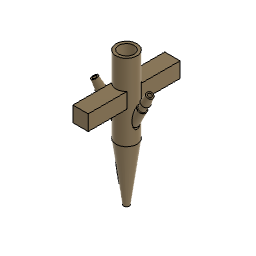
Flush_tool v11 (Autodesk Fusion 360 design; units mm, degrees)
Autodesk Fusion 360 part; units mm, degrees
note: some values were not read from the file. Chosen so that the rebuilt part matches the saved one: where a step starts.
sketch "Sketch1" plane through (0, 0, 0) normal (0, 0, 1) x (1, 0, 0)
  circle A0 centre (0, 0) radius 4
  circle A1 centre (0, 0) radius 5.5
  dimension "d1" = 8
  dimension "d2" = 11
  constraint coincident A0.centre A1.centre
  measures "d1" diameter of A0
  measures "d2" diameter of A1
ref_plane "WorkPlane1" through (0, 0, -15) normal (0, 0, 1) x (1, 0, 0)
sketch "Sketch2" plane through (0, 0, -15) normal (0, 0, 1) x (1, 0, 0)
  circle A0 centre (0, 0) radius 3.45
  dimension "d6" = 6.9
  constraint coincident A0.centre origin
  measures "d6" diameter of A0
extrude "Extrude1" add sketch "Sketch1" against normal blind 40 contours A0 | A1
ref_plane "WorkPlane2" through (0, 0, -70) normal (0, 0, -1) x (-1, 0, 0)
sketch "Sketch3" plane through (0, 0, -70) normal (0, 0, -1) x (-1, 0, 0)
  circle A0 centre (0, 0) radius 1.5
  dimension "d10" = 3
  constraint coincident A0.centre origin
  measures "d10" diameter of A0
loft "Loft1" add profiles "Sketch3" section 1 face at (-1.4907, 0.2732, -40) section 2
ref_plane "WorkPlane3" through (0, 0, 0) normal (0, 1, 0) x (0, 0, 1)
sketch "Sketch4" plane through (0, 0, 0) normal (0, 1, 0) x (1, 0, 0)
  line L0 (0, 0) -> (0, 15) construction
  line L1 (0, 15) -> (4, 15)
  line L2 (0, 15) -> (-4, 15)
  line L3 (-4, 15) -> (-4, 23)
  line L4 (-4, 23) -> (4, 23)
  line L5 (4, 23) -> (4, 15)
  dimension "d12" = 15
  dimension "d13" = 4
  dimension "d14" = 4
  dimension "d15" = 8
  dimension "d16" = 8
  dimension "d17" = 8
  constraint coincident L0.start origin
  constraint vertical L0
  constraint horizontal L1
  constraint perpendicular L0 L2
  constraint perpendicular L2 L3
  constraint perpendicular L3 L4
  constraint perpendicular L4 L5
  measures "d12" distance of L0.start L0.end
  measures "d13" distance of L0.end L1.end
  measures "d14" distance of L0.end L2.end
  measures "d15" distance of L2.end L3.end
  measures "d16" distance of L3.end L4.end
  measures "d17" distance of L4.end L1.end
extrude "Extrude2" add sketch "Sketch4" along normal blind 24 and the other way blind 24
loft "Loft2" cut profiles "Sketch1", "Sketch2" section 1 contours A0 section 2
extrude "Extrude3" cut sketch "Sketch2" against normal blind 3
ref_plane "WorkPlane4" through (0, 0, -28) normal (0, 0, 1) x (1, 0, 0)
sketch "Sketch5" plane through (0, 0, -28) normal (0, 0, 1) x (1, 0, 0)
  circle A0 centre (0, 0) radius 5.5
  line L0 (0, 0) -> (5.5, 0)
  line L1 (0, 0) -> (-4.7631, -2.75)
  line L2 (0, 0) -> (5.5, 0) construction
  line L3 (0, 0) -> (-4.7631, 2.75)
  line L4 (0, 0) -> (5.5, 0) construction
  line L5 (0, 0) -> (4.7631, -2.75) construction
  line L6 (0, 0) -> (5.5, 0) construction
  line L7 (0, 0) -> (4.7631, 2.75) construction
  line L8 (0, 0) -> (5.5, 0) construction
  dimension "d25" = 150
  dimension "d26" = 5.5
  dimension "d27" = 150
  dimension "d28" = 5.5
  dimension "d29" = 5.5
  dimension "d30" = 30
  dimension "d32" = 5.5
  dimension "d33" = 30
  constraint coincident A0.centre L0.start
  constraint coincident A0 L0.end
  constraint horizontal L0
  constraint horizontal L2
  constraint horizontal L4
  constraint horizontal L6
  constraint horizontal L8
  measures "d25" angle of L1 L2
  measures "d26" distance of A0.centre L1.end
  measures "d27" angle of L3 L4
  measures "d28" distance of A0.centre L3.end
  measures "d29" distance of A0.centre L5.end
  measures "d30" angle of L5 L6
  measures "d32" distance of A0.centre L7.end
  measures "d33" angle of L7 L8
ref_plane "WorkPlane5" through (-4.7631, -2.75, -28) normal (-0.5, 0.866025, 0) x (-0.866025, -0.5, 0)
sketch "Sketch6" plane through (0, 0, 0) normal (-0.5, 0.866025, 0) x (-0.866025, -0.5, 0)
  line L0 (-5.5, -40) -> (5.5, -40) construction
  line L1 (-5.5, -40) -> (5.5, -40) construction
  line L2 (1.5, -70) -> (-1.5, -70) construction
  line L3 (5.5, -40) -> (2.5, -40) construction
  line L4 (5.5, -28) -> (2.5, -28) construction
  line L5 (2.5, -28) -> (2.5, -33.991) construction
  line L6 (5.5, -28) -> (2.5, -33.991) construction
  line L7 (2.5, -40) -> (2.5, -33.991) construction
  line L8 (-5.5, -23) -> (-15.4641, -23)
  line L9 (-15.4641, -15) -> (-15.4641, -23)
  line L10 (-5.5, -15) -> (-15.4641, -15)
  line L11 (8.5359, -15) -> (15.4641, -15)
  line L12 (8.5359, -15) -> (5.5, -15)
  line L13 (15.4641, -15) -> (15.4641, -23)
  line L14 (15.4641, -23) -> (8.5359, -23)
  line L15 (8.5359, -23) -> (5.5, -23)
  line L16 (1.5, -70) -> (-1.5, -70)
  line L17 (5.5, 0) -> (-5.5, 0)
  line L18 (1.5, -70) -> (5.5, -40)
  line L19 (-1.5, -70) -> (-5.5, -40)
  line L20 (-5.5, 0) -> (-5.5, -15)
  line L21 (-5.5, -23) -> (-5.5, -40)
  line L22 (5.5, 0) -> (5.5, -15)
  line L23 (5.5, -23) -> (5.5, -40)
  line L24 (5.5, -28) -> (12.2164, -14.5877)
  line L25 (5.5, -28) -> (15.5, -28) construction
  line L26 (5.5, -40) -> (3.3854, -55.8596) construction
  line L27 (2.5, -40) -> (3.3854, -55.8596)
  line L28 (3.3854, -55.8596) -> (3.8313, -63.8472)
  line L29 (4, -30.9955) -> (3.4824, -32.9274)
  line L30 (4, -30.9955) -> (6, -30.9955) construction
  line L31 (3.4824, -32.9274) -> (3.1351, -34.897)
  line L32 (3.4824, -32.9274) -> (5.4748, -32.9274) construction
  line L33 (3.1351, -34.897) -> (2.5, -40)
  line L34 (4, -30.9955) -> (5.5, -28)
  point P0 (5.5, -28)
  point P1 (4, -30.9955)
  point P2 (2.5, -40)
  point P3 (3.1351, -34.897)
  point P4 (3.4824, -32.9274)
  dimension "d34" = 3
  dimension "d35" = 3
  dimension "d36" = 5.991
  dimension "d37" = 63.4
  dimension "d38" = 15
  dimension "d79" = 16
  dimension "d80" = 8
  dimension "d110" = 105
  dimension "d111" = 2
  dimension "d112" = 100
  dimension "d113" = 2
  constraint coincident L0.end L1.end
  constraint parallel L0 L3
  constraint coincident P0 L4.start
  constraint horizontal L4
  constraint perpendicular L4 L5
  constraint horizontal L25
  constraint coincident L18 L26.end
  constraint parallel L27 L28
  constraint midpoint L6 P1
  constraint coincident P2 L3.end
  constraint horizontal L30
  constraint coincident P1 L29.start
  constraint horizontal L32
  constraint coincident P3 L31.end
  constraint coincident P4 L29.end
  measures "d34" distance of L0.end P2
  measures "d35" distance of P0 L4.end
  measures "d36" distance of L4.end L5.end
  measures "d37" angle of L24 L25
  measures "d38" distance of P0 L24.end
  measures "d79" distance of L0.end L26.end
  measures "d80" distance of L26.end L28.end
  measures "d110" angle of L29 L30
  measures "d111" distance of P1 P4
  measures "d112" angle of L31 L32
  measures "d113" distance of P4 P3
pipe "Pipe1" add diameter 4.4 path "Sketch6" along L24 L6 L7 L27 L28 for 0.38 of its length starting at (-10.5797, -6.1082, -14.5877) heading (0.3878, 0.2239, -0.8942)
pipe "Pipe2" cut diameter 2 path "Sketch6" along L24 L34 L29 L31 L33 L27 L28
ref_plane "WorkPlane6" through (4.7631, -2.75, -28) normal (-0.5, -0.866025, 0) x (0.866025, -0.5, 0)
sketch "Sketch7" plane through (0, 0, 0) normal (-0.5, -0.866025, 0) x (0.866025, -0.5, 0)
  ellipse E0 centre (-6.1082, -14.5877) end of major axis (-3.9741, -14.0533) minor radius 0.8531 (-5.5, -13.6201) -> (-8.2502, -15) ccw
  line L0 (-6.2698, -23) -> (-8.5359, -23) construction
  line L1 (-8.2502, -15) -> (-8.5359, -15) construction
  line L2 (-8.5359, -23) -> (-15.4641, -23) construction
  line L3 (-15.4641, -15) -> (-8.5359, -15) construction
  line L4 (15.4641, -15) -> (5.5, -15) construction
  line L5 (-15.4641, -23) -> (-15.4641, -15) construction
  line L6 (15.4641, -23) -> (15.4641, -15) construction
  line L7 (15.4641, -23) -> (5.5, -23) construction
  line L8 (1.5, -70) -> (-1.5, -70) construction
  line L9 (5.5, 0) -> (-5.5, 0) construction
  line L10 (-6.2698, -23) -> (-5.5, -26.0746) construction
  line L11 (1.5, -70) -> (5.5, -40) construction
  line L12 (-1.5, -70) -> (-5.5, -40) construction
  line L13 (-5.5, 0) -> (-5.5, -13.6201) construction
  line L14 (-5.5, -26.0746) -> (-5.5, -40) construction
  line L15 (5.5, 0) -> (5.5, -15) construction
  line L16 (5.5, -23) -> (5.5, -40) construction
  line L17 (-5.5, -28) -> (-2.5, -28) construction
  line L18 (-5.5, -40) -> (-2.5, -40) construction
  line L19 (-2.5, -28) -> (-2.5, -33.991) construction
  line L20 (-5.5, -28) -> (-2.5, -33.991) construction
  line L21 (-2.5, -40) -> (-2.5, -33.991) construction
  line L22 (-5.5, -28) -> (-12.2164, -14.5877)
  line L23 (-5.5, -28) -> (9.5, -28) construction
  line L24 (-5.5, -40) -> (-3.3854, -55.8596) construction
  line L25 (-2.5, -40) -> (-3.3854, -55.8596)
  line L26 (-3.3854, -55.8596) -> (-4.3887, -73.8317)
  line L27 (-4, -30.9955) -> (-3.2235, -33.8933)
  line L28 (-4, -30.9955) -> (-3, -30.9955) construction
  line L29 (-3.2235, -33.8933) -> (-2.8762, -35.8629)
  line L30 (-3.2235, -33.8933) -> (-2.7412, -33.8933) construction
  line L31 (-2.8762, -35.8629) -> (-2.5675, -35.8629) construction
  line L32 (-2.5, -40) -> (-2.5872, -39.0038)
  line L33 (-2.5, -40) -> (-1.5, -40) construction
  line L34 (-2.5872, -39.0038) -> (-2.8762, -35.8629)
  line L35 (-5.5, -28) -> (-4, -30.9955)
  point P0 (-5.5, -28)
  point P1 (-4, -30.9955)
  dimension "d47" = 3
  dimension "d48" = 3
  dimension "d49" = 5.991
  dimension "d52" = 116.6
  dimension "d53" = 15
  dimension "d81" = 16
  dimension "d82" = 18
  dimension "d125" = 75
  dimension "d126" = 3
  dimension "d127" = 80
  dimension "d128" = 2
  dimension "d131" = 95
  dimension "d132" = 1
  constraint coincident P0 L17.start
  constraint perpendicular L14 L17
  constraint coincident L12.end L14.end
  constraint perpendicular L14 L18
  constraint perpendicular L18 L19
  constraint horizontal L23
  constraint coincident L12 L24.end
  constraint parallel L25 L26
  constraint midpoint L20 P1
  constraint horizontal L28
  constraint coincident P1 L27.start
  constraint horizontal L30
  constraint horizontal L31
  constraint horizontal L33
  measures "d47" distance of P0 L17.end
  measures "d48" distance of L12.end L18.end
  measures "d49" distance of L17.end L19.end
  measures "d52" angle of L22 L23
  measures "d53" distance of P0 L22.end
  measures "d81" distance of L12.end L24.end
  measures "d82" distance of L24.end L26.end
  measures "d125" angle of L27 L28
  measures "d126" distance of P1 L27.end
  measures "d127" angle of L29 L30
  measures "d128" distance of L27.end L29.end
  measures "d131" angle of L32 L33
  measures "d132" distance of L18.end L32.end
ref_plane "WorkPlane7" through (0, 0, 0) normal (0, 1, 0) x (0, 0, 1)
sketch "Sketch8" plane through (0, 0, 0) normal (0, 1, 0) x (1, 0, 0)
  ellipse E0 centre (-10.5797, 14.5877) end of major axis (-8.5613, 13.7124) minor radius 0.4925 (-12.5981, 15.463) -> (-8.5613, 13.7124) ccw
  line L0 (-1.5, 70) -> (1.5, 70) construction
  line L1 (-5.5, 0) -> (5.5, 0) construction
  line L2 (-6.7815, 28.8753) -> (-5.5, 31.8304) construction
  line L3 (-8.5613, 13.7124) -> (-5.5, 20.7714) construction
  line L4 (-12.5981, 15.463) -> (-6.7815, 28.8753) construction
  line L5 (-1.5, 70) -> (-5.5, 40) construction
  line L6 (1.5, 70) -> (5.5, 40) construction
  line L7 (5.5, 0) -> (5.5, 40) construction
  line L8 (-5.5, 0) -> (-5.5, 20.7714) construction
  line L9 (-5.5, 31.8304) -> (-5.5, 40) construction
  line L10 (5.5, 28) -> (2.5, 28) construction
  line L11 (5.5, 40) -> (2.5, 40) construction
  line L12 (2.5, 28) -> (2.5, 33.991) construction
  line L13 (5.5, 28) -> (2.5, 33.991) construction
  line L14 (2.5, 40) -> (2.5, 33.991) construction
  line L15 (0, 70) -> (0, 60) construction
  line L16 (5.5, 28) -> (12.2163, 14.5876)
  line L17 (0, 60) -> (0, 61)
  line L18 (4, 30.9955) -> (3.316, 32.8749)
  line L19 (4, 30.9955) -> (4.9934, 30.9955) construction
  line L20 (3.316, 32.8749) -> (2.5395, 35.7727)
  line L21 (3.316, 32.8749) -> (4.658, 32.8749) construction
  line L22 (2.5395, 35.7727) -> (2.0186, 38.7271)
  line L23 (2.5395, 35.7727) -> (4.3992, 35.7727) construction
  line L24 (5.5, 28) -> (4, 30.9955)
  line L25 (0, 60) -> (0.2615, 57.0114)
  line L26 (0, 60) -> (0.9993, 60) construction
  line L27 (0.2615, 57.0114) -> (2.0186, 38.7271)
  point P0 (5.5, 28)
  point P1 (4, 30.9955)
  point P2 (2.5, 40)
  dimension "d63" = 3
  dimension "d64" = 3
  dimension "d65" = 5.991
  dimension "d66" = 10
  dimension "d67" = 15
  dimension "d72" = 1
  dimension "d114" = 110
  dimension "d115" = 2
  dimension "d116" = 105
  dimension "d117" = 3
  dimension "d118" = 100
  dimension "d119" = 3
  dimension "d120" = 85
  dimension "d121" = 3
  constraint coincident P0 L10.start
  constraint perpendicular L7 L10
  constraint coincident L6.end L7.end
  constraint perpendicular L7 L11
  constraint vertical L12
  constraint midpoint L0 L15.start
  constraint perpendicular L0 L15
  constraint parallel L13 L16
  constraint vertical L17
  constraint midpoint L13 P1
  constraint coincident P2 L11.end
  constraint horizontal L19
  constraint coincident P1 L18.start
  constraint horizontal L21
  constraint horizontal L23
  constraint horizontal L26
  measures "d63" distance of P0 L10.end
  measures "d64" distance of L6.end P2
  measures "d65" distance of L10.end L12.end
  measures "d66" distance of L15.start L15.end
  measures "d67" distance of P0 L16.end
  measures "d72" distance of L15.end L17.end
  measures "d114" angle of L18 L19
  measures "d115" distance of P1 L18.end
  measures "d116" angle of L20 L21
  measures "d117" distance of L18.end L20.end
  measures "d118" angle of L22 L23
  measures "d119" distance of L20.end L22.end
  measures "d120" angle of L25 L26
  measures "d121" distance of L15.end L25.end
pipe "Pipe5" add diameter 4.4 path "Sketch8" along L16 L24 L18 L20 L22
pipe "Pipe6" cut diameter 2 path "Sketch8" along L16 L24 L18 L20 L22 L27 L25 L17
ref_plane "WorkPlane8" through (0, 0, -61) normal (0, 0, 1) x (1, 0, 0)
sketch "Sketch9" plane through (0, 0, -61) normal (0, 0, 1) x (1, 0, 0)
  ellipse E0 centre (12.2163, 0) end of major axis (12.2163, -2.2) minor radius 1.9671 (12.2163, -2.2) -> (12.2163, 2.2) ccw
  ellipse E1 centre (-10.5797, -6.1082) end of major axis (-11.6797, -4.2029) minor radius 1.9671 (-11.6797, -4.2029) -> (-9.4797, -8.0134) ccw
  line L0 (4, 3.7749) -> (4, 24)
  line L1 (4, 24) -> (-4, 24)
  line L2 (-4, -24) -> (4, -24)
  line L3 (4, -24) -> (4, -3.7749)
  line L4 (12.2163, 2.2) -> (5.0408, 2.2)
  line L5 (12.2163, -2.2) -> (5.0408, -2.2)
  line L6 (-9.4797, -8.0134) -> (-4, -4.8497)
  line L7 (-11.6797, -4.2029) -> (-5.8631, -0.8447)
  line L8 (-4, 3.7749) -> (-4, 24)
  line L9 (-4, -24) -> (-4, -4.8497)
  arc A0 (4, -3.7749) -> (5.0408, -2.2) centre (0, 0) ccw
  arc A1 (-4, 3.7749) -> (-5.4655, -0.6152) centre (0, 0) ccw
  arc A2 (5.0408, 2.2) -> (4, 3.7749) centre (0, 0) ccw
  line L10 (-5.8631, -0.8447) -> (-5.4655, -0.6152)
  circle A3 centre (0, 0) radius 1
  dimension "d133" = 2
  constraint concentric A0 A3
  measures "d133" diameter of A3
sketch "Sketch10" plane through (0, 0, -70) normal (0, 0, -1) x (-1, 0, 0)
  circle A0 centre (0, 0) radius 1
  dimension "d78" = 2
  constraint coincident A0.centre origin
  measures "d78" diameter of A0
loft "Loft3" cut profiles "Sketch10", "Sketch9" section 1 section 2 contours A3
pipe "Pipe7" add diameter 4.4 path "Sketch7" along L22 L20 L21 L25 L26 for 0.32 of its length starting at (-10.5797, 6.1082, -14.5877) heading (0.3878, -0.2239, -0.8942)
pipe "Pipe8" cut diameter 2 path "Sketch7" along L22 L35 L27 L29 L34 L32 L25 L26
sketch "Sketch11" plane through (0, 0, 0) normal (-0.5, -0.866025, 0) x (0.866025, -0.5, 0)
  spline S0 degree 3 poles (-2.6794, -61.1544) (-2.6797, -61.1512) (-2.6799, -61.148) (-2.6802, -61.1448) (-2.6806, -61.1401) (-2.6811, -61.1337) (-2.6831, -61.109) (-2.6851, -61.0854) (-2.6994, -60.9119) (-2.7186, -60.686) (-2.7637, -60.1702) (-2.7955, -59.8211) (-2.8647, -59.1028) (-2.9021, -58.733) (-3.0205, -57.6192) (-3.1081, -56.8712) (-3.3587, -54.9062) (-3.5879, -53.3688) (-3.8448, -51.8922) (-3.8878, -51.6512) (-3.9729, -51.186) (-4.0153, -50.9604) (-4.0603, -50.7255) (-4.0707, -50.6717) (-4.0823, -50.6114) (-4.0856, -50.5947) (-4.0885, -50.5797) (-4.0891, -50.5767) (-4.0895, -50.5742) (-4.0901, -50.5711) (-4.0907, -50.568) (-4.0914, -50.5649) knots 0.49273 0.49273 0.49273 0.49273 0.495423 0.495423 0.495423 0.499405 0.499405 0.508623 0.508623 0.56814 0.56814 0.671198 0.671198 0.774256 0.774256 0.980372 0.980372 1.368979 1.368979 1.437471 1.437471 1.505962 1.505962 1.525688 1.525688 1.535551 1.535551 1.53841 1.53841 1.53841 1.542008 1.542008 1.542008 1.542008
  line L0 (-13.0398, -15) -> (-10.2492, -13.6026)
  ellipse E0 centre (10.5796, -14.5876) end of major axis (8.5612, -13.7123) minor radius 0.4925 (12.2917, -15) -> (8.5612, -13.7123) ccw
  ellipse E1 centre (-6.1082, -14.5877) end of major axis (-3.9741, -14.0533) minor radius 0.8531 (-5.5, -13.6201) -> (-8.2502, -15) ccw
  line L1 (-8.2502, -15) -> (-8.5359, -15)
  line L2 (-10.4642, -23) -> (-15.4641, -23)
  line L3 (-15.4641, -15) -> (-13.0398, -15)
  line L4 (-9.5495, -15) -> (-8.5359, -15)
  line L5 (15.4641, -15) -> (12.2917, -15)
  line L6 (8.0028, -15) -> (5.5, -15)
  line L7 (-15.4641, -23) -> (-15.4641, -15)
  line L8 (15.4641, -23) -> (15.4641, -15)
  line L9 (15.4641, -23) -> (9.3294, -23)
  line L10 (1.5, -70) -> (-1.5, -70)
  line L11 (5.5, 0) -> (-5.5, 0)
  line L12 (-7.4671, -28.9851) -> (-5.5, -32.9134)
  line L13 (-10.4642, -23) -> (-7.4671, -28.9851)
  line L14 (-10.2492, -13.6026) -> (-9.5495, -15)
  line L15 (8.5612, -13.7123) -> (8.0028, -15)
  line L16 (9.3294, -23) -> (5.528, -31.7659)
  line L17 (1.5, -70) -> (5.5, -40)
  line L18 (-1.5, -70) -> (-2.6794, -61.1544)
  line L19 (-4.0914, -50.5649) -> (-5.5, -40)
  line L20 (-5.5, 0) -> (-5.5, -13.6201)
  line L21 (-5.5, -32.9134) -> (-5.5, -40)
  line L22 (5.5, 0) -> (5.5, -15)
  line L23 (5.5, -31.8546) -> (5.5, -40)
  line L24 (-10.2492, -13.6026) -> (-10.6963, -13.8265)
  line L25 (-10.2492, -13.6026) -> (-8.0105, -18.0734)
  line L26 (-8.0105, -18.0734) -> (-10.6963, -13.8265)
  line L27 (-8.0105, -18.0734) -> (-8.4575, -18.2973)
  line L28 (-8.0105, -18.0734) -> (-6.2194, -21.65)
  line L29 (-6.2194, -21.65) -> (-6.6665, -21.8739)
  line L30 (-8.4575, -18.2973) -> (-6.6665, -21.8739)
  line L31 (5.528, -31.7659) -> (5.5, -31.8546)
  dimension "d91" = 0.5
  dimension "d92" = 5
  dimension "d94" = 0.5
  dimension "d95" = 4
  dimension "d96" = 0.5
  constraint coincident L0.end L14.start
  constraint perpendicular L14 L24
  constraint perpendicular L24 L25
  constraint perpendicular L25 L27
  constraint perpendicular L27 L28
  constraint perpendicular L28 L29
  measures "d91" distance of L0.end L24.end
  measures "d92" distance of L0.end L25.end
  measures "d94" distance of L25.end L27.end
  measures "d95" distance of L25.end L28.end
  measures "d96" distance of L28.end L29.end
revolve "Revolve1" cut sketch "Sketch11" angle 360 about axis through (-4.7631, 2.75, -28) along (-0.387771, 0.22388, 0.894154) contours L0 L14 L24 L25 L26
revolve "Revolve2" cut sketch "Sketch11" angle 360 about axis through (-4.7631, 2.75, -28) along (-0.387771, 0.22388, 0.894154) contours L27 L28 L29 L30
sketch "Sketch12" plane through (0, 0, 0) normal (-0.5, 0.866025, 0) x (-0.866025, -0.5, 0)
  ellipse E0 centre (6.1082, -14.5877) end of major axis (4.4591, -14.1748) minor radius 0.6592 (7.7626, -14.9733) -> (5.5, -13.8304) ccw
  ellipse E1 centre (-10.5796, -14.5876) end of major axis (-8.5612, -13.7123) minor radius 0.4925 (-11.6796, -14.5876) -> (-12.2917, -15) ccw
  ellipse E2 centre (-10.5796, -14.5876) end of major axis (-8.5612, -13.7123) minor radius 0.4925 (-8.5612, -13.7123) -> (-11.6796, -14.5876) ccw
  spline S0 degree 3 poles (3.195, -56.1902) (3.1081, -56.8712) (3.0205, -57.6192) (2.9021, -58.733) (2.8647, -59.1028) (2.7955, -59.8211) (2.7637, -60.1702) (2.7186, -60.686) (2.6994, -60.9119) (2.6851, -61.0854) (2.6831, -61.109) (2.6811, -61.1337) (2.6806, -61.1401) (2.6802, -61.1448) (2.6799, -61.148) (2.6797, -61.1512) (2.6794, -61.1544) knots 0 0 0 0 0.206116 0.206116 0.309175 0.309175 0.412233 0.412233 0.471749 0.471749 0.480968 0.480968 0.484949 0.484949 0.484949 0.487642 0.487642 0.487642 0.487642
  spline S1 degree 3 poles (4.0914, -50.5649) (4.0907, -50.568) (4.0901, -50.5711) (4.0895, -50.5742) (4.0891, -50.5767) (4.0885, -50.5797) (4.0856, -50.5947) (4.0823, -50.6114) (4.0707, -50.6717) (4.0603, -50.7255) (4.0153, -50.9604) (3.9729, -51.186) (3.8878, -51.6512) (3.8448, -51.8922) (3.5879, -53.3688) (3.3587, -54.9062) (3.195, -56.1902) knots 1.54882 1.54882 1.54882 1.54882 1.552417 1.552417 1.552417 1.555277 1.555277 1.56514 1.56514 1.584865 1.584865 1.653357 1.653357 1.721849 1.721849 2.110455 2.110455 2.110455 2.110455
  line L0 (12.2164, -14.5877) -> (13.0398, -15)
  line L1 (10.2492, -13.6026) -> (12.2164, -14.5877)
  line L2 (-9.3294, -23) -> (-15.4641, -23)
  line L3 (-15.4641, -15) -> (-15.4641, -23)
  line L4 (-5.5, -15) -> (-8.0028, -15)
  line L5 (-12.2917, -15) -> (-15.4641, -15)
  line L6 (8.5359, -15) -> (9.5495, -15)
  line L7 (13.0398, -15) -> (15.4641, -15)
  line L8 (8.5359, -15) -> (7.7589, -15)
  line L9 (15.4641, -15) -> (15.4641, -23)
  line L10 (15.4641, -23) -> (10.4642, -23)
  line L11 (1.5, -70) -> (-1.5, -70)
  line L12 (5.5, 0) -> (-5.5, 0)
  line L13 (7.7626, -14.9733) -> (7.7589, -15)
  line L14 (-9.3294, -23) -> (-5.528, -31.7659)
  line L15 (-8.5612, -13.7123) -> (-8.0028, -15)
  line L16 (7.4671, -28.9851) -> (5.5, -32.9134)
  line L17 (10.2492, -13.6026) -> (9.5495, -15)
  line L18 (10.4642, -23) -> (7.4671, -28.9851)
  line L19 (1.5, -70) -> (2.6794, -61.1544)
  line L20 (4.0914, -50.5649) -> (5.5, -40)
  line L21 (-1.5, -70) -> (-5.5, -40)
  line L22 (-5.5, 0) -> (-5.5, -15)
  line L23 (-5.5, -31.8546) -> (-5.5, -40)
  line L24 (5.5, 0) -> (5.5, -13.8304)
  line L25 (5.5, -32.9134) -> (5.5, -40)
  line L26 (10.2492, -13.6026) -> (10.6963, -13.8265)
  line L27 (10.2492, -13.6026) -> (8.0105, -18.0734)
  line L28 (10.6963, -13.8265) -> (8.0105, -18.0734)
  line L29 (8.0105, -18.0734) -> (6.2194, -21.65)
  line L30 (6.2194, -21.65) -> (6.6665, -21.8739)
  line L31 (8.0105, -18.0734) -> (8.4575, -18.2973)
  line L32 (6.6665, -21.8739) -> (8.4575, -18.2973)
  line L33 (-5.528, -31.7659) -> (-5.5, -31.8546)
  dimension "d98" = 0.5
  dimension "d99" = 5
  dimension "d100" = 4
  dimension "d101" = 0.5
  dimension "d102" = 0.5
  constraint coincident L1.start L17.start
  constraint perpendicular L17 L26
  constraint perpendicular L1 L27
  constraint parallel L27 L29
  constraint perpendicular L29 L30
  constraint perpendicular L29 L31
  measures "d98" distance of L1.start L26.end
  measures "d99" distance of L1.start L27.end
  measures "d100" distance of L27.end L29.end
  measures "d101" distance of L29.end L30.end
  measures "d102" distance of L27.end L31.end
revolve "Revolve3" cut sketch "Sketch12" angle 360 about axis through (-4.7631, -2.75, -28) along (-0.387771, -0.22388, 0.894154) contours L29 L30 L31 L32 | L1 L17 L26 L27 L28
sketch "Sketch13" plane through (0, 0, 0) normal (0, 1, 0) x (1, 0, 0)
  ellipse E0 centre (-10.5797, 14.5877) end of major axis (-12.1394, 15.2641) minor radius 0.3806 (-12.1424, 15.2559) -> (-9.2633, 13.8265) ccw
  ellipse E1 centre (-10.5797, 14.5877) end of major axis (-12.1394, 15.2641) minor radius 0.3806 (-9.2633, 13.8265) -> (-9.0239, 13.9035) ccw
  ellipse E2 centre (-8.6408, 19.0585) end of major axis (-6.6225, 18.1831) minor radius 0.4925 (-6.6275, 18.173) -> (-6.9568, 18.6689) ccw
  ellipse E3 centre (-8.6408, 19.0585) end of major axis (-6.6225, 18.1831) minor radius 0.4925 (-10.0761, 20.0217) -> (-10.6632, 19.9232) ccw
  ellipse E4 centre (-7.0898, 22.6351) end of major axis (-5.0714, 21.7598) minor radius 0.4925 (-9.1081, 23.5104) -> (-8.7738, 23.0246) ccw
  ellipse E5 centre (-7.0898, 22.6351) end of major axis (-5.0714, 21.7598) minor radius 0.4925 (-5.6545, 21.6719) -> (-5.5, 21.6546) ccw
  line L0 (14.1834, 15.5727) -> (10.2491, 13.6026)
  line L1 (-1.5, 70) -> (1.5, 70)
  line L2 (-5.5, 0) -> (5.5, 0)
  line L3 (-9.0239, 13.9035) -> (-6.6275, 18.173)
  line L4 (-12.1424, 15.2559) -> (-10.6632, 19.9232)
  line L5 (-8.7738, 23.0246) -> (-10.0761, 20.0217)
  line L6 (-5.6545, 21.6719) -> (-6.9568, 18.6689)
  line L7 (14.1834, 15.5727) -> (6.0239, 31.8671)
  line L8 (10.2491, 13.6026) -> (5.5, 23.0866)
  line L9 (-6.7815, 28.8753) -> (-5.5, 31.8304)
  line L10 (-9.1081, 23.5104) -> (-6.7815, 28.8753)
  line L11 (-1.5, 70) -> (-5.5, 40)
  line L12 (1.5, 70) -> (5.5, 40)
  line L13 (5.5, 0) -> (5.5, 23.0866)
  line L14 (5.5, 33.3067) -> (5.5, 40)
  line L15 (-5.5, 0) -> (-5.5, 21.6546)
  line L16 (-5.5, 31.8304) -> (-5.5, 40)
  line L17 (14.1834, 15.5727) -> (13.7363, 15.3488)
  line L18 (14.1834, 15.5727) -> (11.9447, 20.0435)
  line L19 (13.7363, 15.3488) -> (11.9447, 20.0435)
  line L20 (11.9447, 20.0435) -> (11.4976, 19.8196)
  line L21 (11.9447, 20.0435) -> (10.1537, 23.6201)
  line L22 (10.1537, 23.6201) -> (9.7066, 23.3962)
  line L23 (11.4976, 19.8196) -> (9.7066, 23.3962)
  line L24 (6.0239, 31.8671) -> (5.5, 33.3067)
  dimension "d104" = 0.5
  dimension "d105" = 5
  dimension "d106" = 0.5
  dimension "d107" = 4
  dimension "d108" = 0.5
  constraint coincident L0.start L7.start
  constraint perpendicular L7 L17
  constraint perpendicular L17 L18
  constraint perpendicular L18 L20
  constraint coincident L7 L21.end
  constraint perpendicular L21 L22
  measures "d104" distance of L0.start L17.end
  measures "d105" distance of L0.start L18.end
  measures "d106" distance of L18.end L20.end
  measures "d107" distance of L18.end L21.end
  measures "d108" distance of L21.end L22.end
revolve "Revolve4" cut sketch "Sketch13" angle 360 about axis through (5.5, 0, -28) along (0.447751, 0, 0.894158) contours L0 L7 L17 L18 L19 | L7 L20 L21 L22 L23
equation "d1 = Pipette_Large_Diameter"
equation "Pipette_Large_Diameter = 8 mm"
equation "Pipette_Small_Diameter = 6.9 mm"
equation "d6 = Pipette_Small_Diameter"
equation "d25 = angles"
equation "d27 = angles"
equation "d30 = 180 deg - angles"
equation "angles = 150 deg"
equation "d33 = 180 deg - angles"
equation "d52 = 180 deg - 63.4 deg"
